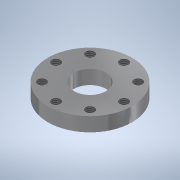
# Autodesk Inventor part: FreeHorn
Saved by Autodesk Inventor 2020.4 (Build 244396000, 396)
## iProperties
Created: 2015-11-22
Part Number: FreeHorn
Material: アルミニウム 6061
Document SubType Name: Modeling
Designer: haya
Density: 2.7 g/cm^3
Appearance: アルミニウム - ダーク
Mass: 2.533 g
Surface Area: 10.4083 cm^2
Volume: 0.938147 cm^3
Description: 既製品
Author: haya
Autodesk Inventor part; units mm, degrees
ref_plane "YZ Plane" through (0, 0, 0) normal (1, 0, 0) x (0, 1, 0)
ref_plane "XZ Plane" through (0, 0, 0) normal (0, 1, 0) x (-1, 0, 0)
ref_plane "XY Plane" through (0, 0, 0) normal (0, 0, 1) x (1, 0, 0)
sketch "スケッチ1" plane through (0, 0, 0) normal (0, 0, 1) x (1, 0, 0)
  circle A0 centre (0, 0) radius 10.5
  circle A1 centre (0, 0) radius 4
  dimension "d0" = 21
  dimension "d1" = 8
  constraints: 2 centre point, 2 coincident
  measures "d0" diameter of A0
  measures "d1" diameter of A1
extrude "押し出し1" add sketch "スケッチ1" along normal blind 3.5
sketch "スケッチ2" plane through (0, 0, 3.5) normal (0, 0, 1) x (1, 0, 0)
  line L0 (0, 0) -> (0, 10.5) construction
  circle A0 centre (0, 0) radius 10.5 projected
  point P0 (0, 8.5)
  point P1 (-6.0104, 6.0104)
  point P2 (-8.5, 0)
  point P3 (-6.0104, -6.0104)
  point P4 (0, -8.5)
  point P5 (6.0104, -6.0104)
  point P6 (8.5, 0)
  point P7 (6.0104, 6.0104)
  dimension "d4" = 8.5
  dimension "d7" = 360
  constraints: 2 end point, 1 point on line, 1 vertical, 1 vertical alignment, 10 other
  measures "d4" distance of point (0, 8.5) L0.start
hole "穴1" at (0, 8.5, 3.5) at (-6.0104, 6.0104, 3.5) at (-8.5, 0, 3.5) at (-6.0104, -6.0104, 3.5) at (0, -8.5, 3.5) at (6.0104, -6.0104, 3.5) at (8.5, 0, 3.5) at (6.0104, 6.0104, 3.5) direction (0, 0, -1) diameter 2.113 end through all thread size "M2.6x0.45" class "6H" standard "ISO Metric profile"
